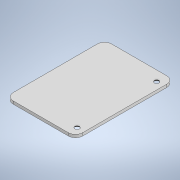
# Autodesk Inventor part: Krishka
Saved by Autodesk Inventor 2021.2 (Build 252289000, 289)
## iProperties
Created: 2022-01-13
Part Number: Krishka
Material: Типовые
Document SubType Name: Modeling
Designer: Иваныч
Density: 1 g/cm^3
Appearance: По умолчанию
Author: Иваныч
Autodesk Inventor part; units mm, degrees
ref_plane "YZ Plane" through (0, 0, 0) normal (1, 0, 0) x (0, 1, 0)
ref_plane "XZ Plane" through (0, 0, 0) normal (0, 1, 0) x (-1, 0, 0)
ref_plane "XY Plane" through (0, 0, 0) normal (0, 0, 1) x (1, 0, 0)
sketch "Эскиз1" plane through (0, 0, 0) normal (0, 1, 0) x (-1, 0, 0)
  line L0 (26.0474, 33.1003) -> (-11.9526, 33.1003)
  line L1 (-16.9526, 28.1003) -> (-16.9526, -29.8997)
  line L2 (-11.9526, -34.8997) -> (26.0474, -34.8997)
  line L3 (31.0474, -29.8997) -> (31.0474, 28.1003)
  arc A0 (31.0474, 28.1003) -> (26.0474, 33.1003) centre (26.0474, 28.1003) ccw
  arc A1 (-11.9526, 33.1003) -> (-16.9526, 28.1003) centre (-11.9526, 28.1003) ccw
  arc A2 (-16.9526, -29.8997) -> (-11.9526, -34.8997) centre (-11.9526, -29.8997) ccw
  arc A3 (26.0474, -34.8997) -> (31.0474, -29.8997) centre (26.0474, -29.8997) ccw
  point P0 (0, 0)
  dimension "d0" = 68
  dimension "d1" = 48
  dimension "d2" = 5
  constraints: 8 end point, 8 point on circle, 8 tangent, 4 centre point, 3 equal radius, 2 parallel, 1 horizontal, 1 perpendicular
  measures "d0" distance between parallel lines of L0 L2
  measures "d1" distance between parallel lines of L3 L1
  measures "d2" radius of A0
extrude "Выдавливание1" add sketch "Эскиз1" along normal blind 2
sketch "Эскиз2" plane through (0, 0, 0) normal (0, -1, 0) x (1, 0, 0)
  circle A0 centre (12.0526, -27.8997) radius 1.6
  line L0 (11.9526, -34.8997) -> (-26.0474, -34.8997) projected
  line L1 (16.9526, 28.1003) -> (16.9526, -29.8997) projected
  circle A1 centre (12.0526, 27.1003) radius 1.6
  line L2 (-26.0474, 33.1003) -> (11.9526, 33.1003) projected
  point P0 (0, 0)
  dimension "d7" = 7
  dimension "d9" = 4.9
  dimension "d13" = 4.9
  dimension "d14" = 6
  constraints: 2 centre point
  measures "d7" distance from line of A0.centre L0
  measures "d9" distance from line of A0.centre L1
  measures "d13" distance from line of L1 A1.centre
  measures "d14" distance from line of L2 A1.centre
extrude "Выдавливание2" cut sketch "Эскиз2" against normal blind 10
chamfer "Фаска1" distance 2 angle 45 2 edges at (10.4526, 0, 27.1003) (10.4526, 0, -27.8997)
